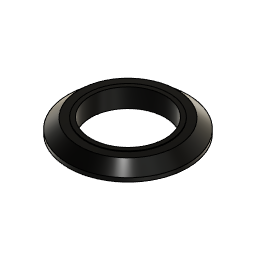
NMJ nut washer (Autodesk Fusion 360 design; units mm, degrees)
Autodesk Fusion 360 part; units mm, degrees
sketch "Sketch1" plane through (0, 0, 0) normal (0, 1, 0) x (1, 0, 0)
  line L0 (0, 0) -> (4.95, 0) construction
  line L1 (4.95, 0) -> (5.5, 0)
  line L2 (5.5, 0) -> (5.5, -0.63)
  line L3 (4.95, 0) -> (4.95, -2.5)
  line L4 (5.5, -0.63) -> (7.95, -0.63)
  line L5 (0, 0) -> (0, -2.6) construction
  line L6 (4.95, -2.5) -> (5.5, -2.5)
  line L7 (5.5, -2.5) -> (5.5, -2.4)
  line L8 (5.5, -2.4) -> (6.5, -2.4)
  line L9 (7.95, -0.63) -> (7.95, -1.13)
  line L10 (6.5, -2.4) -> (7.95, -1.13)
  dimension "d1" = 4.95
  dimension "d2" = 0.55
  dimension "d3" = 0.63
  dimension "d6" = 3
  dimension "d7" = 0.55
  dimension "d8" = 0.1
  dimension "d9" = 1.55
  dimension "d10" = 0.5
  dimension "d11" = 2.5
  constraint coincident L0.start L5.start
  constraint horizontal L0
  constraint parallel L0 L1
  constraint perpendicular L1 L2
  constraint perpendicular L0 L3
  constraint perpendicular L2 L4
  constraint perpendicular L0 L5
  constraint perpendicular L3 L6
  constraint perpendicular L6 L7
  constraint perpendicular L7 L8
  constraint perpendicular L4 L9
  measures "d1" distance of L0.start L0.end
  measures "d2" distance of L0.end L1.end
  measures "d3" distance of L1.end L2.end
  measures "d6" distance of L3 L4.end
  measures "d7" distance of L3.end L6.end
  measures "d8" distance of L6.end L7.end
  measures "d9" distance of L3 L8.end
  measures "d10" distance of L4.end L9.end
  measures "d11" distance of L0.end L3.end
revolve "Revolve1" add sketch "Sketch1" angle 360 about axis through (0, 0, 0) along (0, 0, 1)
equation "d1 = ( 9.9 / 2 ) * 1 mm"
